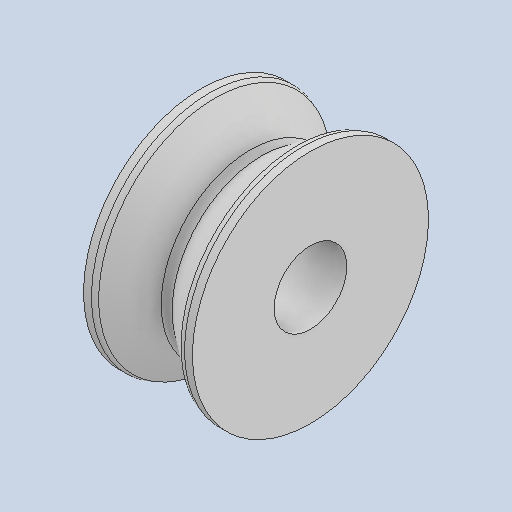
# Autodesk Inventor part: uxcell_V624ZZ_4mmx13mmx6mm
Saved by Autodesk Inventor 2025.3 (Build 293356030, 356C)
## iProperties
Created: 2025-09-01
Part Number: uxcell_V624ZZ_4mmx13mmx6mm
Material: Generic
Document SubType Name: Modeling
Designer: tvoko
Density: 1 g/cm^3
Appearance: Default
Author: tvoko
Autodesk Inventor part; units mm, degrees
ref_plane "YZ Plane" through (0, 0, 0) normal (1, 0, 0) x (0, 1, 0)
ref_plane "XZ Plane" through (0, 0, 0) normal (0, 1, 0) x (-1, 0, 0)
ref_plane "XY Plane" through (0, 0, 0) normal (0, 0, 1) x (1, 0, 0)
sketch "Sketch1" plane through (0, 0, 0) normal (0, 0, 1) x (1, 0, 0)
  line L0 (0, 0) -> (6, 0) construction
  line L1 (0, 2) -> (6, 2)
  line L2 (3, 2) -> (3, 0) construction
  line L3 (0, 2) -> (0, 6.5)
  line L4 (0, 6.5) -> (0.6, 6.5)
  line L5 (0.6, 6.5) -> (3, 4.7)
  line L6 (3, 4.7) -> (5.4, 6.5)
  line L7 (5.4, 6.5) -> (6, 6.5)
  line L8 (6, 6.5) -> (6, 2)
  line L9 (0.6, 6.5) -> (5.4, 6.5) construction
  line L10 (3, 6.5) -> (3, 2) construction
  dimension "d0" = 6
  dimension "d1" = 6.5
  dimension "d2" = 2
  dimension "d3" = 4.8
  dimension "d4" = 1.8
  constraints: 22 end point, 4 perpendicular, 4 point on line, 3 horizontal, 3 midpoint, 1 vertical
  measures "d0" distance between parallel lines of L8 L3
  measures "d1" distance between parallel lines of L0 L4
  measures "d2" distance of L2.start L2.end
  measures "d3" distance of L6.end L4.end
  measures "d4" distance from line of L5.end L9
revolve "Revolution1" add sketch "Sketch1" angle 360 about axis through (0, 0, 0) along (1, 0, 0)
fillet "Fillet1" radius 0.5 3 edges at (3, -4.7, 0) (0.6, -6.5, 0) (5.4, -6.5, 0)
body "Solid1"
